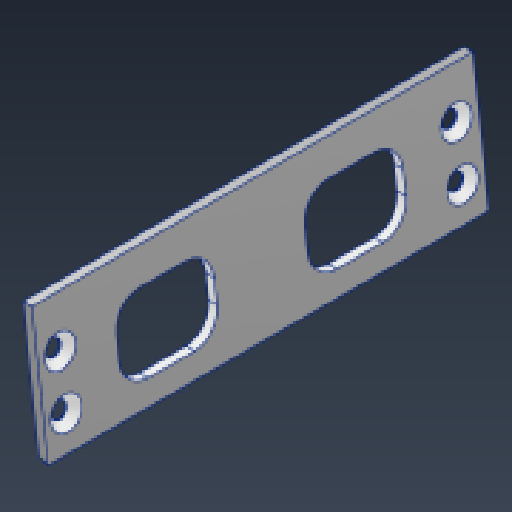
# Autodesk Inventor part: front-plate
Saved by Autodesk Inventor 2023 (Build 270158000, 158)
## iProperties
Created: 2025-04-06
Part Number: front-plate
Material: Aluminum 6061
Document SubType Name: Modeling
Designer: szymo
Density: 2.7 g/cm^3
Appearance: Aluminum - Flat
Mass: 11.7631 g
Surface Area: 52.9722 cm^2
Volume: 4.35671 cm^3
Author: szymo
Autodesk Inventor part; units mm, degrees
ref_plane "YZ Plane" through (0, 0, 0) normal (1, 0, 0) x (0, 1, 0)
ref_plane "XZ Plane" through (0, 0, 0) normal (0, 1, 0) x (-1, 0, 0)
ref_plane "XY Plane" through (0, 0, 0) normal (0, 0, 1) x (1, 0, 0)
sketch "Sketch1" plane through (0, 0, 0) normal (0, 0, 1) x (1, 0, 0)
  line L0 (-4.7358, 33.5983) -> (-1.1571, 4.4523) projected
  line L1 (-6.7497, 33.5894) -> (-4.7358, 33.5983) projected
  line L2 (-3.2634, 5.1955) -> (-6.7497, 33.5894) projected
  line L3 (-1.1571, 4.4523) -> (-3.2634, 5.1955) projected
  line L4 (-4.3471, -2.4575) -> (4.3462, -4.7869) projected
  line L5 (4.3462, -4.7869) -> (-0.9571, 4.3987) projected
  line L6 (-0.9571, 4.3987) -> (-2.406, 4.7869) projected
  line L7 (-2.406, 4.7869) -> (-4.3471, -2.4575) projected
  point P0 (0, 0)
ref_plane "Work Plane1" through (-4.3892, -4.8255, -99) normal (0, 0, -1) x (0, 1, 0)
extrude "Extrusion1" add sketch "Sketch1" against normal up to surface (99 mm away) contours L0 L3 L2 L1
ref_plane "Work Plane2" through (8.5183, 16.2258, -28.325) normal (0.9999901, 0.0044406, 0) x (0, 0, -1)
sketch "Sketch2" plane through (8.5183, 16.2258, -28.325) normal (0.9999901, 0.0044406, 0) x (0, 0, -1)
  line L0 (-10.495, 4.15) -> (-10.495, -0.85)
  line L1 (10.495, 4.15) -> (10.495, -0.85)
  line L2 (31.855, 4.15) -> (31.855, -0.85)
  line L3 (52.845, 4.15) -> (52.845, -0.85)
  line L4 (-10.495, -0.85) -> (10.495, -0.85) construction
  line L5 (31.855, -0.85) -> (52.845, -0.85) construction
  circle A0 centre (-5.245, -0.85) radius 5.25
  circle A1 centre (5.245, -0.85) radius 5.25
  circle A2 centre (37.105, -0.85) radius 5.25
  circle A3 centre (47.595, -0.85) radius 5.25
  line L6 (-5.245, 4.15) -> (5.2802, 4.15)
  line L7 (-5.245, -6.1) -> (5.245, -6.1)
  line L8 (37.105, -6.1) -> (47.595, -6.1)
  line L9 (37.105, 4.15) -> (47.595, 4.15)
  arc A4 (0, 4.3791) -> (0, 3.9209) centre (-5.245, 4.15) ccw projected
  arc A5 (0, 3.9209) -> (0, 4.3791) centre (5.245, 4.15) ccw projected
  arc A6 (42.35, 3.9209) -> (42.35, 4.3791) centre (47.595, 4.15) ccw projected
  arc A7 (42.35, 4.3791) -> (42.35, 3.9209) centre (37.105, 4.15) ccw projected
  line L10 (-10.495, 4.15) -> (10.495, 4.15) construction
  line L11 (31.855, 4.15) -> (52.845, 4.15) construction
  line L12 (-5.245, -0.85) -> (-5.245, 4.15) construction
  line L13 (5.245, 4.15) -> (5.245, -0.85) construction
  line L14 (37.105, 4.15) -> (37.105, -0.85) construction
  line L15 (47.595, 4.15) -> (47.595, -0.85) construction
  line L16 (-5.245, 9.4) -> (5.245, 9.4)
  line L17 (37.105, 9.4) -> (47.595, 9.4)
  arc A8 (-5.245, 9.9) -> (-10.995, 4.15) centre (-5.245, 4.15) ccw
  arc A9 (10.995, 4.15) -> (5.245, 9.9) centre (5.245, 4.15) ccw
  arc A10 (5.245, -6.6) -> (10.995, -0.85) centre (5.245, -0.85) ccw
  arc A11 (-10.995, -0.85) -> (-5.245, -6.6) centre (-5.245, -0.85) ccw
  line L18 (-10.995, -0.85) -> (-10.995, 4.15)
  line L19 (-5.245, -6.6) -> (5.245, -6.6)
  line L20 (-5.245, 9.9) -> (5.245, 9.9)
  line L21 (10.995, -0.85) -> (10.995, 4.15)
  line L22 (-5.245, -0.85) -> (-5.245, -6.6) construction
  arc A12 (37.105, 9.9) -> (31.355, 4.15) centre (37.105, 4.15) ccw
  arc A13 (53.345, 4.15) -> (47.595, 9.9) centre (47.595, 4.15) ccw
  arc A14 (47.595, -6.6) -> (53.345, -0.85) centre (47.595, -0.85) ccw
  arc A15 (31.355, -0.85) -> (37.105, -6.6) centre (37.105, -0.85) ccw
  line L23 (31.355, 4.15) -> (31.355, -0.85)
  line L24 (37.105, -6.6) -> (47.595, -6.6)
  line L25 (53.345, -0.85) -> (53.345, 4.15)
  line L26 (47.595, 9.9) -> (37.105, 9.9)
  line L27 (47.595, -0.85) -> (47.595, -6.6) construction
  point P0 (-28.325, -16.1878)
  point P1 (31.855, -0.85)
  point P2 (52.845, -0.85)
  point P3 (42.35, -0.6209)
  point P4 (42.35, -1.0791)
  point P5 (0, -1.0791)
  point P6 (0, -0.6209)
  point P7 (10.495, -0.85)
  point P8 (-10.495, -0.85)
  point P9 (45.9942, 4.15)
  point P10 (38.7058, 4.15)
  point P11 (3.6442, 4.15)
  point P12 (-3.6442, 4.15)
  point P13 (52.845, 4.15)
  point P14 (31.855, 4.15)
  point P15 (10.495, 4.15)
  point P16 (-10.495, 4.15)
  dimension "d4" = 5
  dimension "d5" = 5
  dimension "d6" = 5
  dimension "d7" = 5
  dimension "d19" = 0.5
  dimension "d20" = 0.5
  constraints: 56 end point, 22 point on circle, 22 point on line, 15 vertical, 10 coincident, 9 horizontal, 8 centre point, 4 equal length, 1 perpendicular, 1 tangent, 16 other
  measures "d4" distance of L0.start L0.end
  measures "d5" distance of L1.start L1.end
  measures "d6" distance of L2.start L2.end
  measures "d7" distance of L3.start L3.end
  measures "d19" distance between parallel lines of L20 L16
  measures "d20" distance between parallel lines of L26 L17
extrude "Extrusion2" cut sketch "Sketch2" against normal through all contours A4 A0 L0 | A4 A5 A1 L6 A0 | A0 A4 A1 | L16 A5 A4 | A0 A4 | A0 A1 L7 | L6 A1 A5 A4 A0 | A4 A5 A1 A0 | A1 A0 | A0 A1 A5 | L1 A1 A5 | A1 A5 | A7 A2 L2 | A7 A6 A3 L9 A2 | A2 A7 A3 | L17 A6 A7 | A2 A7 | A2 A3 L8 | L9 A3 A6 A7 A2 | A7 A6 A3 A2 | A3 A2 | A2 A3 A6 | L3 A3 A6 | A3 A6 | L20 A9 L21 A10 L19 A11 L18 A8 | L26 A13 L25 A14 L24 A15 L23 A12
sketch "Sketch3" plane through (-4.7358, 33.5983, 0) normal (0.9925462, 0.1218693, 0) x (0, 0, -1)
  circle A0 centre (5, -10.615) radius 2.3 projected
  circle A1 centre (5, -22.115) radius 2.3 projected
  line L0 (0, -28.5569) -> (0, -6.7854) projected
  line L1 (0, -28.5569) -> (10, -28.5569) projected
  line L2 (10, -6.7854) -> (10, -28.5569) projected
  line L3 (0, -6.7854) -> (10, -6.7854) projected
  line L4 (49.5, -12.1831) -> (49.5, -16.4876)
  point P0 (0, -33.9251)
  point P1 (94, -10.615)
  point P2 (94, -22.115)
  dimension "d17" = 49.5
  constraints: 2 coincident, 2 end point, 2 symmetric about line, 1 vertical
  measures "d17" distance between parallel lines of L4 L0
hole "Hole1" at (-3.4422, 23.0625, -5) at (-2.0407, 11.6482, -5) at (-3.4422, 23.0625, -94) at (-2.0407, 11.6482, -94) direction (-0.9925462, -0.1218693, 0) diameter 3.6 depth 5 countersink diameter 7 countersink angle 90 clearance for "Countersunk Flat Head Screw ISO 2009/7046" size "M3" standard "ISO"
body "Solid1"
